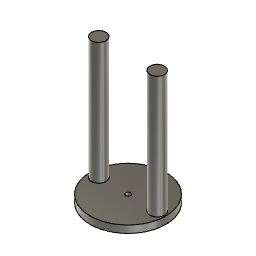
Fiber stack depressor v2 (Autodesk Fusion 360 design; units mm, degrees)
Autodesk Fusion 360 part; units mm, degrees
sketch "Sketch1" plane through (0, 0, 0) normal (0, 0, 1) x (1, 0, 0)
  circle A0 centre (0, 0) radius 15.5
  circle A1 centre (0, 0) radius 1
  dimension "d1" = 31
  dimension "d2" = 2
  constraint coincident A0.centre A1.centre
  constraint concentric A0 A1
  measures "d1" diameter of A0
  measures "d2" diameter of A1
extrude "Extrude1" add sketch "Sketch1" along normal blind 3
sketch "Sketch2" plane through (0, 0, 3) normal (0, 0, 1) x (-1, 0, 0)
  circle A0 centre (0, 0) radius 1
  circle A1 centre (0, 0) radius 15.5
  circle A2 centre (12, 0) radius 3
  circle A3 centre (-12, 0) radius 3
  line L0 (15.5, 0) -> (12, 0)
  line L1 (-12, 0) -> (-15.5, 0)
  dimension "d7" = 6
  constraint equal A2 A3
  constraint coincident A1 L0.start
  constraint coincident A2.centre L0.end
  constraint horizontal L0
  constraint coincident A3.centre L1.start
  constraint coincident A1 L1.end
  constraint horizontal L1
  constraint equal L0 L1
  measures "d7" diameter of A2
extrude "Extrude2" add sketch "Sketch2" along normal blind 50 contours A2 | A3
